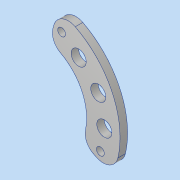
# Autodesk Inventor part: gearboxBearingHolderForward
Saved by Autodesk Inventor 2017.3 (Build 213256000, 256)
## iProperties
Created: 2018-09-02
Part Number: gearboxBearingHolderForward
Material: Aluminum 6061
Document SubType Name: Modeling
Designer: Derek Wider
Density: 2.7 g/cm^3
Appearance: Aluminum - Flat
Author: Derek Wider
Autodesk Inventor part; units mm, degrees
ref_plane "YZ Plane" through (0, 0, 0) normal (1, 0, 0) x (0, 1, 0)
ref_plane "XZ Plane" through (0, 0, 0) normal (0, 1, 0) x (-1, 0, 0)
ref_plane "XY Plane" through (0, 0, 0) normal (0, 0, 1) x (1, 0, 0)
sketch "Sketch2" plane through (0, 0, 0) normal (0, 0, 1) x (1, 0, 0)
  circle A0 centre (28.194, 0) radius 3.175
  circle A1 centre (25.645, 11.7147) radius 3.175
  circle A2 centre (17.397, 20.4153) radius 3.175
  line L0 (0, 0) -> (28.194, 0) construction
  line L1 (25.645, 11.7147) -> (0, 0) construction
  line L2 (17.397, 20.4153) -> (0, 0) construction
  line L3 (18.663, -9.1026) -> (31.2762, -15.2544)
  line L4 (5.1766, 20.1089) -> (8.6751, 33.6993)
  arc A3 (18.663, -9.1026) -> (5.1766, 20.1089) centre (0, 0) ccw
  arc A4 (31.2762, -15.2544) -> (8.6751, 33.6993) centre (0, 0) ccw
  circle A5 centre (10.2574, 26.1255) radius 1.651
  circle A6 centre (26.5379, -9.1377) radius 1.651
  line L5 (10.2574, 26.1255) -> (0, 0) construction
  line L6 (0, 0) -> (26.5379, -9.1377) construction
  dimension "d2" = 6.35
  dimension "d4" = 28.194
  dimension "d5" = 26.8224
  dimension "d6" = 11.9888
  dimension "d7" = 11.9888
  dimension "d9" = 41.529
  dimension "d11" = 69.596
  dimension "d14" = 28.067
  dimension "d15" = 19
  dimension "d16" = 19
  dimension "d17" = 7
  dimension "d18" = 7
  dimension "d19" = 3.302
  constraints: 14 end point, 7 centre point, 4 line through centre, 4 point on circle, 3 equal radius, 2 coincident, 2 equal length, 1 horizontal
  measures "d2" diameter of A0
  measures "d4" distance of L0.start L0.end
  measures "d5" distance of L2.start L0.start
  measures "d6" distance of L1.start L0.end
  measures "d7" distance of L1.start L2.start
  measures "d9" diameter of A3
  measures "d11" diameter of A4
  measures "d14" distance of L5.start L5.end
  measures "d15" angle of L2 L5
  measures "d16" angle of L0 L6
  measures "d17" angle of L5 L4
  measures "d18" angle of L6 L3
  measures "d19" diameter of A5
extrude "Extrusion1" add sketch "Sketch2" along normal blind 3.175
fillet "Fillet1" radius 6.35 4 edges at (8.6751, 33.6993, 1.5875) (5.1766, 20.1089, 1.5875) (18.663, -9.1026, 1.5875) (31.2762, -15.2544, 1.5875)
body "Solid1"
